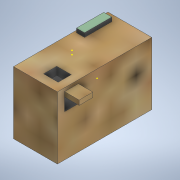
# Autodesk Inventor part: Atas
Saved by Autodesk Inventor 2021 (Build 250183000, 183)
## iProperties
Created: 2021-12-07
Part Number: Atas
Material: Generic
Document SubType Name: Modeling
Designer: LENOVO
Density: 1 g/cm^3
Appearance: Default
Author: LENOVO
Autodesk Inventor part; units mm, degrees
ref_plane "YZ Plane" through (0, 0, 0) normal (1, 0, 0) x (0, 1, 0)
ref_plane "XZ Plane" through (0, 0, 0) normal (0, 1, 0) x (-1, 0, 0)
ref_plane "XY Plane" through (0, 0, 0) normal (0, 0, 1) x (1, 0, 0)
sketch "Sketch1" plane through (0, 0, 0) normal (0, 1, 0) x (-1, 0, 0)
  line L0 (7.1862, 13.3676) -> (-7.8138, 13.3676)
  line L1 (-7.8138, 13.3676) -> (-7.8138, -19.1776)
  line L2 (-7.8138, -19.1776) -> (7.1862, -19.1776)
  line L3 (7.1862, -19.1776) -> (7.1862, 13.3676)
  point P0 (0, 0)
  dimension "d0" = 15
  constraints: 8 end point, 2 parallel, 1 horizontal, 1 perpendicular
  measures "d0" distance of L2.end L1.end
extrude "Extrusion1" add sketch "Sketch1" along normal blind 3
sketch "Sketch2" plane through (0, 3, 0) normal (0, 1, 0) x (1, 0, 0)
  line L0 (0.84, -11.5857) -> (6.3178, -11.5857)
  line L1 (6.3178, -11.5857) -> (6.3178, -6.6455)
  line L2 (6.3178, -6.6455) -> (0.84, -6.6455)
  line L3 (0.84, -6.6455) -> (0.84, -11.5857)
  point P0 (0, 0)
  constraints: 8 end point, 2 parallel, 1 horizontal, 1 perpendicular
extrude "Extrusion2" cut sketch "Sketch2" against normal blind 4.5
sketch "Sketch3" plane through (0, 3, 0) normal (0, 1, 0) x (1, 0, 0)
  line L0 (-6.4027, 18.2927) -> (-3.3498, 18.2927)
  line L1 (-3.3498, 18.2927) -> (-3.3498, 8.0094)
  line L2 (-3.3498, 8.0094) -> (-6.4027, 8.0094)
  line L3 (-6.4027, 8.0094) -> (-6.4027, 18.2927)
  point P0 (0, 0)
  constraints: 8 end point, 2 parallel, 1 horizontal, 1 perpendicular
extrude "Extrusion3" add sketch "Sketch3" along normal blind 1.5
sketch "Sketch4" plane through (-7.1862, 0, 13.3676) normal (0, 0, 1) x (1, 0, 0)
  line L0 (0, 3) -> (15, 3) projected
  line L1 (0, 3) -> (15, 3)
  line L2 (15, 3) -> (15, -19.0502)
  line L3 (15, -19.0502) -> (0, -19.0502)
  line L4 (0, -19.0502) -> (0, 3)
  point P0 (7.1862, 0)
  constraints: 8 end point, 2 parallel, 1 horizontal, 1 perpendicular
extrude "Extrusion4" add sketch "Sketch4" along normal blind 1.5
sketch "Sketch5" plane through (-7.1862, 0, 13.3676) normal (0, 0, -1) x (-1, 0, 0)
  line L0 (-15, -19.0502) -> (-15, 0) projected
  line L1 (0, 0) -> (0, -19.0502) projected
  line L2 (-15, -6.2009) -> (0, -6.2009)
  line L3 (0, -6.2009) -> (0, -4.8004)
  line L4 (0, -4.8004) -> (-15, -4.8004)
  line L5 (-15, -4.8004) -> (-15, -6.2009)
  point P0 (-7.1862, 0)
  constraints: 8 end point, 2 parallel, 2 point on line, 1 horizontal, 1 perpendicular
extrude "Extrusion5" add sketch "Sketch5" along normal blind 32.5
sketch "Sketch6" plane through (7.8138, 0, -19.1776) normal (0, 0, -1) x (-1, 0, 0)
  line L0 (0, 0) -> (0, 3) projected
  line L1 (15, -6.2009) -> (15, -19.0502) projected
  line L2 (0, 3) -> (15, 3)
  line L3 (15, 3) -> (15, -19.0502)
  line L4 (15, -19.0502) -> (0, -19.0502)
  line L5 (0, -19.0502) -> (0, 3)
  point P0 (7.8138, 0)
  constraints: 8 end point, 2 parallel, 1 horizontal, 1 perpendicular
extrude "Extrusion6" add sketch "Sketch6" along normal blind 1.5
sketch "Sketch7" plane through (-7.1862, -19.0502, -19.1776) normal (0, -1, 0) x (1, 0, 0)
  line L0 (15, -1.5) -> (15, 34.0452) projected
  line L1 (15, -1.5) -> (0, -1.5)
  line L2 (0, -1.5) -> (0, 34.0452)
  line L3 (0, 34.0452) -> (15, 34.0452)
  line L4 (15, 34.0452) -> (15, -1.5)
  point P0 (7.1862, 19.1776)
  constraints: 8 end point, 2 parallel, 1 horizontal, 1 perpendicular
extrude "Extrusion7" add sketch "Sketch7" along normal blind 1.5
sketch "Sketch8" plane through (0, 3, 0) normal (0, 1, 0) x (1, 0, 0)
  point P0 (0, 0)
sketch "Sketch10" plane through (7.8138, 3, 14.8676) normal (1, 0, 0) x (0, 0, -1)
  line L0 (0, 0) -> (35.5452, 0) projected
  line L1 (35.5452, 0) -> (35.5452, -23.5502) projected
  line L2 (0, 0) -> (35.5452, 0)
  line L3 (35.5452, 0) -> (35.5452, -23.5502)
  line L4 (35.5452, -23.5502) -> (0, -23.5502)
  line L5 (0, -23.5502) -> (0, 0)
  point P0 (14.8676, -3)
  constraints: 8 end point, 2 parallel, 1 horizontal, 1 perpendicular
extrude "Extrusion9" add sketch "Sketch10" along normal blind 1.5
sketch "Sketch11" plane through (9.3138, 3, 14.8676) normal (1, 0, 0) x (0, 0, -1)
  point P0 (14.8676, -3)
sketch "Sketch12" plane through (9.3138, 3, 14.8676) normal (1, 0, 0) x (0, 0, -1)
  line L0 (1.5, -7.8004) -> (34, -7.8004) projected
  line L1 (2.6857, -1.2569) -> (7.8665, -1.2569)
  line L2 (7.8665, -1.2569) -> (7.8665, -7.8004)
  line L3 (7.8665, -7.8004) -> (2.6857, -7.8004)
  line L4 (2.6857, -7.8004) -> (2.6857, -1.2569)
  point P0 (14.8676, -3)
  point P1 (2.6857, -7.8004)
  constraints: 8 end point, 2 parallel, 1 horizontal, 1 perpendicular, 1 point on line
extrude "Extrusion10" cut sketch "Sketch12" against normal blind 1.5
sketch "Sketch13" plane through (-7.1862, -19.0502, -19.1776) normal (0, 1, 0) x (1, 0, 0)
  line L0 (11.8023, -6.3584) -> (1.3351, -6.3584)
  line L1 (1.3351, -6.3584) -> (1.3351, -31.4677)
  line L2 (1.3351, -31.4677) -> (11.8023, -31.4677)
  line L3 (11.8023, -31.4677) -> (11.8023, -6.3584)
  point P0 (7.1862, -19.1776)
  constraints: 8 end point, 2 parallel, 1 horizontal, 1 perpendicular
extrude "Extrusion11" add sketch "Sketch13" along normal blind 1
sketch "Sketch14" plane through (-7.1862, -18.0502, -19.1776) normal (0, 1, 0) x (1, 0, 0)
  line L0 (10.9591, -8.0288) -> (2.1896, -8.0288)
  line L1 (2.1896, -8.0288) -> (2.1896, -30.8703)
  line L2 (2.1896, -30.8703) -> (10.9591, -30.8703)
  line L3 (10.9591, -30.8703) -> (10.9591, -8.0288)
  point P0 (7.1862, -19.1776)
  constraints: 8 end point, 2 parallel, 1 horizontal, 1 perpendicular
extrude "Extrusion12" add sketch "Sketch14" along normal blind 1
sketch "Sketch15" plane through (-7.1862, -4.8004, 13.3676) normal (0, 1, 0) x (1, 0, 0)
  line L0 (12.3187, 15.0671) -> (8.4438, 15.0671)
  line L1 (8.4438, 15.0671) -> (8.4438, 7.8611)
  line L2 (8.4438, 7.8611) -> (12.3187, 7.8611)
  line L3 (12.3187, 7.8611) -> (12.3187, 15.0671)
  point P0 (7.1862, 13.3676)
  constraints: 8 end point, 2 parallel, 1 horizontal, 1 perpendicular
extrude "Extrusion13" add sketch "Sketch15" along normal blind 1
sketch "Sketch17" plane through (-7.1862, -17.0502, -19.1776) normal (0, 1, 0) x (1, 0, 0)
  line L0 (8.3336, -13.5877) -> (3.2144, -13.5877)
  line L1 (3.2144, -13.5877) -> (3.2144, -29.2984)
  line L2 (3.2144, -29.2984) -> (8.3336, -29.2984)
  line L3 (8.3336, -29.2984) -> (8.3336, -13.5877)
  point P0 (7.1862, -19.1776)
  constraints: 8 end point, 2 parallel, 1 horizontal, 1 perpendicular
extrude "Extrusion15" add sketch "Sketch17" along normal blind 1
sketch "Sketch19" plane through (7.8138, 3, 14.8676) normal (1, 0, 0) x (0, 0, -1)
  line L0 (2.6857, -1.2569) -> (7.8665, -1.2569) projected
  line L1 (7.8665, -1.2569) -> (7.8665, -7.8004) projected
  line L2 (2.6857, -1.2569) -> (7.8665, -1.2569)
  line L3 (7.8665, -1.2569) -> (7.8665, -3)
  line L4 (7.8665, -3) -> (2.6857, -3)
  line L5 (2.6857, -3) -> (2.6857, -1.2569)
  point P0 (14.8676, -3)
  constraints: 8 end point, 2 parallel, 1 horizontal, 1 perpendicular, 1 point on line
extrude "Extrusion16" add sketch "Sketch19" along normal blind 7
sketch "Sketch20" plane through (-7.1862, -4.8004, 13.3676) normal (0, 1, 0) x (1, 0, 0)
  point P0 (7.1862, 13.3676)
sketch "Sketch21" plane through (-7.1862, -4.8004, 13.3676) normal (0, 1, 0) x (1, 0, 0)
  point P0 (7.1862, 13.3676)
sketch "Sketch22" plane through (-7.1862, -4.8004, 13.3676) normal (0, 1, 0) x (1, 0, 0)
  point P0 (7.1862, 13.3676)
sketch "Sketch23" plane through (-7.1862, -4.8004, 13.3676) normal (0, 1, 0) x (1, 0, 0)
  circle A0 centre (11.5182, 22.6981) radius 2.5447
  point P0 (7.1862, 13.3676)
  constraints: 1 centre point
extrude "Extrusion17" cut sketch "Sketch23" against normal blind 1.5
sketch "Sketch24" plane through (-7.1862, -4.8004, 13.3676) normal (0, 1, 0) x (1, 0, 0)
  point P0 (7.1862, 13.3676)
sketch "Sketch25" plane through (-7.1862, -4.8004, 13.3676) normal (0, 1, 0) x (1, 0, 0)
  point P0 (7.1862, 13.3676)
sketch "Sketch26" plane through (-7.1862, -4.8004, 13.3676) normal (0, 1, 0) x (1, 0, 0)
  point P0 (7.1862, 13.3676)
sketch "Sketch27" plane through (-7.1862, -4.8004, 13.3676) normal (0, 1, 0) x (1, 0, 0)
  line L0 (10.9591, 1.6749) -> (10.9591, 24.5164) projected
  circle A0 centre (10.9591, 4.3668) radius 1.0997
  point P0 (7.1862, 13.3676)
  constraints: 1 centre point, 1 point on line
extrude "Extrusion18" cut sketch "Sketch27" against normal blind 1.5
sketch "Sketch28" plane through (0, 4.5, 0) normal (0, 1, 0) x (1, 0, 0)
  point P0 (0, 0)
body "Solid1"
